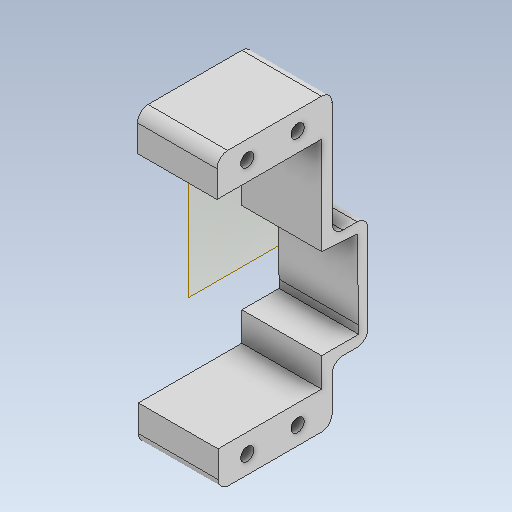
# Autodesk Inventor part: bracket
Saved by Autodesk Inventor 2020 (Build 240168000, 168)
## iProperties
Created: 2019-05-07
Part Number: bracket
Material: Generic
Document SubType Name: Modeling
Designer: erwin
Density: 1 g/cm^3
Appearance: Default
Author: erwin
Autodesk Inventor part; units mm, degrees
ref_plane "XZ Plane" through (0, 0, 0) normal (0, 1, 0) x (-1, 0, 0)
ref_plane "XY Plane" through (0, 0, 0) normal (0, 0, 1) x (1, 0, 0)
ref_plane "Work Plane1" through (-15.5, 0, 0) normal (1, 0, 0) x (0, 1, 0)
sketch "Sketch1" plane through (-15.5, 0, 0) normal (1, 0, 0) x (0, 1, 0)
  line L0 (-0.5, 0) -> (-0.5, -6.716667)
  line L1 (-0.5, -6.716667) -> (-15.5, -6.716667)
  line L2 (-17, -7) -> (-15.5, -7)
  line L3 (-17, 0) -> (-17, -7)
  line L4 (-17, 0) -> (-22.45, 0)
  line L5 (-22.45, 0) -> (-22.45, 19.5)
  line L6 (-22.45, 19.5) -> (-29.45, 19.5)
  line L7 (-29.45, 19.5) -> (-29.45, -2)
  line L8 (-29.45, -2) -> (-19, -2)
  line L9 (-19, -2) -> (-19, -8.716667)
  line L10 (-19, -8.716667) -> (1.5, -8.716667)
  line L11 (-17, -7) -> (-0.5, -7) construction
  line L12 (-9.247706, -7) -> (-9.247706, -16.201099) construction
  line L13 (1.5, -8.716667) -> (1.5, -2)
  line L14 (1.5, -2) -> (25.35, -2)
  line L15 (25.35, -2) -> (25.35, 19.691667)
  line L16 (25.35, 19.691667) -> (18.35, 19.691667)
  line L17 (18.35, 19.691667) -> (18.35, 0)
  line L18 (18.35, 0) -> (0, 0)
  line L19 (-14.45, -1.808333) -> (-14.45, -5.115) construction
  dimension "d1" = 19.5
  dimension "d2" = 2
  dimension "d3" = 2
  dimension "d4" = 2
  dimension "d5" = 7
  dimension "d6" = 7
  dimension "d7" = 2
  dimension "d8" = 8
  dimension "d9" = 40.8
  constraints: 28 end point, 11 perpendicular, 2 horizontal, 2 vertical, 4 other
  measures "d1" distance of L4.end L5.end
  measures "d2" distance between parallel lines of L1 L10
  measures "d3" distance between parallel lines of L3 L9
  measures "d4" distance between parallel lines of L4 L8
  measures "d5" distance of L5.end L6.end
  measures "d6" distance of L15.end L16.end
  measures "d7" distance between parallel lines of L0 L13
  measures "d8" distance between parallel lines of L5 L19
  measures "d9" distance between parallel lines of L17 L5
sketch "Sketch1 outline for Extrusion1" plane through (-15.5, 0, 0) normal (1, 0, 0) x (0, 1, 0)
  line L0 (-17, 0) -> (-22.45, 0)
  line L1 (-17, -7) -> (-17, 0)
  line L2 (-15.5, -7) -> (-17, -7)
  line L3 (-0.5, -6.716667) -> (-15.5, -7)
  line L4 (0, 0) -> (-0.5, -6.716667)
  line L5 (18.35, 0) -> (0, 0)
  line L6 (18.35, 19.691667) -> (18.35, 0)
  line L7 (25.35, 19.691667) -> (18.35, 19.691667)
  line L8 (25.35, -2) -> (25.35, 19.691667)
  line L9 (1.5, -2) -> (25.35, -2)
  line L10 (1.5, -8.716667) -> (1.5, -2)
  line L11 (-19, -8.716667) -> (1.5, -8.716667)
  line L12 (-19, -2) -> (-19, -8.716667)
  line L13 (-29.45, -2) -> (-19, -2)
  line L14 (-29.45, 19.5) -> (-29.45, -2)
  line L15 (-22.45, 19.5) -> (-29.45, 19.5)
  line L16 (-22.45, 0) -> (-22.45, 19.5)
extrude "Extrusion1" add sketch "Sketch1 outline for Extrusion1" along normal blind 15
sketch "Sketch2" plane through (-0.5, 0, 0) normal (1, 0, 0) x (0, 0, -1)
  line L0 (0, -17) -> (0, -22.45)
  line L1 (0, 18.35) -> (0, 0)
  line L2 (-19.5, -29.45) -> (2, -29.45)
  line L3 (2, 25.35) -> (-19.691667, 25.35)
  point P0 (-4.5, -26.05)
  point P1 (-14, -26.05)
  point P2 (-4.5, 21.95)
  point P3 (-14, 21.95)
  dimension "d12" = 4.5
  dimension "d13" = 9.5
  dimension "d14" = 4.5
  dimension "d15" = 9.5
  dimension "d16" = 48
  dimension "d17" = 3.4
  dimension "d18" = 3.4
  measures "d12" distance from line of L0 point (-4.5, -26.05)
  measures "d13" distance of point (-14, -26.05) point (-4.5, -26.05)
  measures "d14" distance from line of L1 point (-4.5, 21.95)
  measures "d15" distance of point (-4.5, 21.95) point (-14, 21.95)
  measures "d16" distance of point (-4.5, 21.95) point (-4.5, -26.05)
  measures "d17" distance from line of L2 point (-4.5, -26.05)
  measures "d18" distance from line of L3 point (-4.5, 21.95)
hole "Hole1" at (-0.5, -26.05, 4.5) at (-0.5, -26.05, 14) at (-0.5, 21.95, 4.5) at (-0.5, 21.95, 14) direction (-1, 0, 0) diameter 2.5 end through all
fillet "Fillet1" radius 2 8 edges at (-8, 25.35, 19.6917) (-8, 25.35, -2) (-8, 1.5, -2) (-8, 1.5, -8.7167) (-8, -19, -8.7167) (-8, -29.45, -2) (-8, -29.45, 19.5) (-8, -19, -2)
equation "\"d2\" = d3"
equation "\"d4\" = d3"
equation "\"d7\" = d3"
equation "\"d14\" = d12"
equation "\"d15\" = d13"
equation "\"d18\" = d17"
body "Solid1"
